Autodesk Inventor part; units mm, degrees
(part 2 of 2)
sketch "Sketch14" plane through (0, 0, 0) normal (-1, 0, 0) x (0, 0, 1)
  line L0 (-10.4499, -187.9273) -> (8.7669, -187.9273) construction
  line L1 (8.7669, -187.9273) -> (8.7669, -196.7101) construction
  line L2 (8.7669, -196.7101) -> (-10.4499, -196.7101) construction
  line L3 (-10.4499, -196.7101) -> (-10.4499, -187.9273) construction
  line L4 (-23.4175, -195.887) -> (-20.8486, -188.267)
  line L5 (-20.8486, -188.267) -> (-19.6013, -188.267)
  line L6 (-19.6013, -188.267) -> (-17.0325, -195.887)
  line L7 (-17.0325, -195.887) -> (-18.1008, -195.887)
  line L8 (-18.1008, -195.887) -> (-18.7924, -193.7566)
  line L9 (-18.7924, -193.7566) -> (-21.7008, -193.7566)
  line L10 (-21.7008, -193.7566) -> (-22.3924, -195.887)
  line L11 (-22.3924, -195.887) -> (-23.4175, -195.887)
  line L12 (-19.0702, -192.8921) -> (-20.2497, -189.3044)
  line L13 (-20.2497, -189.3044) -> (-21.4229, -192.8921)
  line L14 (-21.4229, -192.8921) -> (-19.0702, -192.8921)
  line L15 (-10.4128, -195.887) -> (-11.7281, -195.887)
  line L16 (-11.7281, -195.887) -> (-14.1364, -192.855)
  line L17 (-14.1364, -192.855) -> (-15.2973, -192.855)
  line L18 (-15.2973, -192.855) -> (-15.2973, -195.887)
  line L19 (-15.2973, -195.887) -> (-16.31, -195.887)
  line L20 (-16.31, -195.887) -> (-16.31, -188.267)
  line L21 (-16.31, -188.267) -> (-14.3463, -188.267)
  spline S0 degree 2 poles (-14.3463, -188.267) (-13.6918, -188.267) (-12.8087, -188.409) (-12.4074, -188.6683) knots 0 0 0 1 2 2 2
  spline S1 degree 2 poles (-12.4074, -188.6683) (-12.006, -188.9277) (-11.5429, -189.7366) (-11.5429, -190.3356) knots 0 0 0 1 2 2 2
  spline S2 degree 2 poles (-11.5429, -190.3356) (-11.5429, -191.1692) (-12.395, -192.2993) (-13.1237, -192.571) knots 0 0 0 1 2 2 2
  line L22 (-13.1237, -192.571) -> (-10.4128, -195.887)
  spline S3 degree 2 poles (-12.5988, -190.4159) (-12.5988, -190.0824) (-12.8334, -189.5699) (-13.0804, -189.4032) knots 0 0 0 1 2 2 2
  spline S4 degree 2 poles (-13.0804, -189.4032) (-13.2966, -189.2612) (-13.8708, -189.1438) (-14.2907, -189.1438) knots 0 0 0 1 2 2 2
  line L23 (-14.2907, -189.1438) -> (-15.2973, -189.1438)
  line L24 (-15.2973, -189.1438) -> (-15.2973, -192.009)
  line L25 (-15.2973, -192.009) -> (-14.4081, -192.009)
  spline S5 degree 2 poles (-14.4081, -192.009) (-13.9696, -192.009) (-13.2719, -191.8547) (-13.031, -191.6138) knots 0 0 0 1 2 2 2
  spline S6 degree 2 poles (-13.031, -191.6138) (-12.8087, -191.4039) (-12.5988, -190.8111) (-12.5988, -190.4159) knots 0 0 0 1 2 2 2
  line L26 (-8.0293, -195.887) -> (-8.0293, -189.1685)
  line L27 (-8.0293, -189.1685) -> (-10.5857, -189.1685)
  line L28 (-10.5857, -189.1685) -> (-10.5857, -188.267)
  line L29 (-10.5857, -188.267) -> (-4.4601, -188.267)
  line L30 (-4.4601, -188.267) -> (-4.4601, -189.1685)
  line L31 (-4.4601, -189.1685) -> (-7.0166, -189.1685)
  line L32 (-7.0166, -189.1685) -> (-7.0166, -195.887)
  line L33 (-7.0166, -195.887) -> (-8.0293, -195.887)
  spline S7 degree 2 poles (-1.564, -196.0228) (-2.3914, -196.0228) (-3.5524, -195.677) (-4.0649, -195.43) knots 0 0 0 1 2 2 2
  line L34 (-4.0649, -195.43) -> (-4.0649, -194.158)
  line L35 (-4.0649, -194.158) -> (-3.9908, -194.158)
  spline S8 degree 2 poles (-3.9908, -194.158) (-3.4906, -194.6273) (-2.2247, -195.146) (-1.6381, -195.146) knots 0 0 0 1 2 2 2
  spline S9 degree 2 poles (-1.6381, -195.146) (-0.7983, -195.146) (0.06, -194.4482) (0.06, -193.8739) knots 0 0 0 1 2 2 2
  spline S10 degree 2 poles (0.06, -193.8739) (0.06, -193.417) (-0.3907, -192.8489) (-0.8786, -192.7068) knots 0 0 0 1 2 2 2
  spline S11 degree 2 poles (-0.8786, -192.7068) (-1.2305, -192.608) (-1.8172, -192.4722) (-2.2556, -192.361) knots 0 0 0 1 2 2 2
  spline S12 degree 2 poles (-2.2556, -192.361) (-2.6508, -192.256) (-3.2745, -191.9411) (-3.5153, -191.6879) knots 0 0 0 1 2 2 2
  spline S13 degree 2 poles (-3.5153, -191.6879) (-3.75, -191.4348) (-4.0093, -190.7555) (-4.0093, -190.3109) knots 0 0 0 1 2 2 2
  spline S14 degree 2 poles (-4.0093, -190.3109) (-4.0093, -189.3847) (-2.5643, -188.1311) (-1.4467, -188.1311) knots 0 0 0 1 2 2 2
  spline S15 degree 2 poles (-1.4467, -188.1311) (-0.8045, -188.1311) (0.3317, -188.3843) (0.8196, -188.6251) knots 0 0 0 1 2 2 2
  line L36 (0.8196, -188.6251) -> (0.8196, -189.8354)
  line L37 (0.8196, -189.8354) -> (0.7455, -189.8354)
  spline S16 degree 2 poles (0.7455, -189.8354) (0.3811, -189.502) (-0.7551, -189.008) (-1.3787, -189.008) knots 0 0 0 1 2 2 2
  spline S17 degree 2 poles (-1.3787, -189.008) (-2.0827, -189.008) (-2.9534, -189.6687) (-2.9534, -190.2059) knots 0 0 0 1 2 2 2
  spline S18 degree 2 poles (-2.9534, -190.2059) (-2.9534, -190.6876) (-2.4408, -191.2619) (-1.9592, -191.3915) knots 0 0 0 1 2 2 2
  spline S19 degree 2 poles (-1.9592, -191.3915) (-1.6381, -191.478) (-0.7057, -191.7003) (-0.3969, -191.7929) knots 0 0 0 1 2 2 2
  spline S20 degree 2 poles (-0.3969, -191.7929) (0.3873, -192.0337) (1.116, -193.0032) (1.116, -193.7134) knots 0 0 0 1 2 2 2
  spline S21 degree 2 poles (1.116, -193.7134) (1.116, -194.1641) (0.7516, -195.0286) (0.4244, -195.3312) knots 0 0 0 1 2 2 2
  spline S22 degree 2 poles (0.4244, -195.3312) (0.06, -195.6647) (-0.8662, -196.0228) (-1.564, -196.0228) knots 0 0 0 1 2 2 2
  line L38 (4.7222, -193.0156) -> (1.8385, -193.0156)
  line L39 (1.8385, -193.0156) -> (1.8385, -192.0893)
  line L40 (1.8385, -192.0893) -> (4.7222, -192.0893)
  line L41 (4.7222, -192.0893) -> (4.7222, -193.0156)
  line L42 (10.3662, -195.887) -> (5.951, -195.887)
  line L43 (5.951, -195.887) -> (5.951, -188.267)
  line L44 (5.951, -188.267) -> (6.9637, -188.267)
  line L45 (6.9637, -188.267) -> (6.9637, -194.9854)
  line L46 (6.9637, -194.9854) -> (10.3662, -194.9854)
  line L47 (10.3662, -194.9854) -> (10.3662, -195.887)
  spline S23 degree 2 poles (14.275, -195.2818) (14.1577, -195.3683) (13.7625, -195.677) (13.5772, -195.7696) knots 0 0 0 1 2 2 2
  spline S24 degree 2 poles (13.5772, -195.7696) (13.324, -195.9055) (12.8486, -196.0475) (12.4163, -196.0475) knots 0 0 0 1 2 2 2
  spline S25 degree 2 poles (12.4163, -196.0475) (12.0643, -196.0475) (11.4283, -195.782) (11.1875, -195.5412) knots 0 0 0 1 2 2 2
  spline S26 degree 2 poles (11.1875, -195.5412) (10.959, -195.3065) (10.6811, -194.6149) (10.6811, -194.2321) knots 0 0 0 1 2 2 2
  spline S27 degree 2 poles (10.6811, -194.2321) (10.6811, -193.6393) (11.1813, -192.7995) (11.7247, -192.5586) knots 0 0 0 1 2 2 2
  spline S28 degree 2 poles (11.7247, -192.5586) (12.2063, -192.3363) (13.5155, -192.1696) (14.275, -192.1264) knots 0 0 0 1 2 2 2
  line L48 (14.275, -192.1264) -> (14.275, -191.9411)
  spline S29 degree 2 poles (14.275, -191.9411) (14.275, -191.6077) (14.0712, -191.1939) (13.886, -191.0766) knots 0 0 0 1 2 2 2
  spline S30 degree 2 poles (13.886, -191.0766) (13.7007, -190.9593) (13.1697, -190.8852) (12.8856, -190.8852) knots 0 0 0 1 2 2 2
  spline S31 degree 2 poles (12.8856, -190.8852) (12.5522, -190.8852) (11.6506, -191.0828) (11.1998, -191.2742) knots 0 0 0 1 2 2 2
  line L49 (11.1998, -191.2742) -> (11.1442, -191.2742)
  line L50 (11.1442, -191.2742) -> (11.1442, -190.2924)
  spline S32 degree 2 poles (11.1442, -190.2924) (11.4098, -190.2183) (12.404, -190.033) (12.8918, -190.033) knots 0 0 0 1 2 2 2
  spline S33 degree 2 poles (12.8918, -190.033) (13.4846, -190.033) (14.2935, -190.2183) (14.6146, -190.4591) knots 0 0 0 1 2 2 2
  spline S34 degree 2 poles (14.6146, -190.4591) (14.9295, -190.6938) (15.2383, -191.4409) (15.2383, -191.9782) knots 0 0 0 1 2 2 2
  line L51 (15.2383, -191.9782) -> (15.2383, -195.887)
  line L52 (15.2383, -195.887) -> (14.275, -195.887)
  line L53 (14.275, -195.887) -> (14.275, -195.2818)
  line L54 (14.275, -194.4791) -> (14.275, -192.8921)
  spline S35 degree 2 poles (14.275, -192.8921) (13.9292, -192.923) (12.8856, -193.0279) (12.5583, -193.1267) knots 0 0 0 1 2 2 2
  spline S36 degree 2 poles (12.5583, -193.1267) (12.1755, -193.2441) (11.6753, -193.7319) (11.6753, -194.1641) knots 0 0 0 1 2 2 2
  spline S37 degree 2 poles (11.6753, -194.1641) (11.6753, -194.6581) (12.231, -195.1583) (12.7621, -195.1583) knots 0 0 0 1 2 2 2
  spline S38 degree 2 poles (12.7621, -195.1583) (13.2129, -195.1583) (13.9539, -194.7693) (14.275, -194.4791) knots 0 0 0 1 2 2 2
  spline S39 degree 2 poles (21.3825, -192.9353) (21.3825, -194.337) (20.024, -196.0475) (18.9989, -196.0475) knots 0 0 0 1 2 2 2
  spline S40 degree 2 poles (18.9989, -196.0475) (18.5358, -196.0475) (17.875, -195.819) (17.5539, -195.6214) knots 0 0 0 1 2 2 2
  line L55 (17.5539, -195.6214) -> (17.4922, -195.887)
  line L56 (17.4922, -195.887) -> (16.5906, -195.887)
  line L57 (16.5906, -195.887) -> (16.5906, -187.9273)
  line L58 (16.5906, -187.9273) -> (17.5539, -187.9273)
  line L59 (17.5539, -187.9273) -> (17.5539, -190.7679)
  spline S41 degree 2 poles (17.5539, -190.7679) (17.9183, -190.4406) (18.7642, -190.0083) (19.3015, -190.0083) knots 0 0 0 1 2 2 2
  spline S42 degree 2 poles (19.3015, -190.0083) (20.271, -190.0083) (21.3825, -191.5583) (21.3825, -192.9353) knots 0 0 0 1 2 2 2
  spline S43 degree 2 poles (20.3883, -193.0094) (20.3883, -191.9843) (19.7646, -190.9222) (19.073, -190.9222) knots 0 0 0 1 2 2 2
  spline S44 degree 2 poles (19.073, -190.9222) (18.684, -190.9222) (17.8812, -191.2927) (17.5539, -191.5768) knots 0 0 0 1 2 2 2
  line L60 (17.5539, -191.5768) -> (17.5539, -194.8557)
  spline S45 degree 2 poles (17.5539, -194.8557) (17.9183, -195.0348) (18.4802, -195.183) (18.8136, -195.183) knots 0 0 0 1 2 2 2
  spline S46 degree 2 poles (18.8136, -195.183) (19.5485, -195.183) (20.3883, -194.1394) (20.3883, -193.0094) knots 0 0 0 1 2 2 2
  point P0 (0, 0)
  constraints: 2 other
emboss "Emboss2" sketch "Sketch14" operation cut depth 2.54 direction (1, 0, 0)
sketch "Sketch15" plane through (0, -213.7841, 48.4212) normal (0, 0, 1) x (1, 0, 0)
  line L0 (21.59, 0) -> (21.59, 261.366) projected
  line L1 (17.272, 162.687) -> (21.59, 162.687)
  line L2 (21.59, 162.687) -> (21.59, 170.688)
  line L3 (21.59, 170.688) -> (17.272, 170.688)
  line L4 (17.272, 170.688) -> (17.272, 162.687)
  line L5 (21.59, 264.541) -> (0, 264.541) projected
  point P0 (0, 213.7841)
  point P1 (19.431, 170.688)
  dimension "d78" = 8.001
  dimension "d79" = 4.318
  dimension "d83" = 101.854
  constraints: 8 end point, 2 parallel, 1 horizontal, 1 midpoint, 1 perpendicular, 1 point on line
  measures "d78" distance of L3.end L1.start
  measures "d79" distance between parallel lines of L0 L4
  measures "d83" distance between parallel lines of L5 L1
extrude "Extrusion9" cut sketch "Sketch15" against normal blind 6.35
sketch "Sketch18" plane through (0, -216.9591, -50.0038) normal (0, -1, 0) x (1, 0, 0)
  line L0 (21.59, 43.2816) -> (21.59, 53.2892)
  line L1 (21.59, 53.2892) -> (20.3708, 53.2892)
  line L2 (20.3708, 53.2892) -> (18.6182, 51.2892)
  line L3 (18.6182, 45.2816) -> (18.6182, 51.2892)
  line L4 (21.59, 98.425) -> (0, 98.425) projected
  line L5 (21.59, 95.25) -> (21.59, 0) projected
  line L6 (21.59, 43.2816) -> (20.3708, 43.2816)
  line L7 (20.3708, 43.2816) -> (18.6182, 45.2816)
  point P0 (20.9804, 53.2892)
  dimension "d91" = 1.2192
  dimension "d92" = 2
  dimension "d94" = 6.0076
  dimension "d95" = 10.0076
  dimension "d98" = 1.7526
  dimension "d99" = 0
  dimension "d165" = 45.1358
  constraints: 12 end point, 1 horizontal, 1 midpoint
  measures "d91" distance of L0.end L1.end
  measures "d92" vertical distance of L1.end L2.end
  measures "d94" distance of L3.start L2.end
  measures "d95" distance of L0.start L0.end
  measures "d98" distance from line of L1.end L3
  measures "d99" distance between parallel lines of L5 L0
  measures "d165" distance from line of L4 point (20.98, 53.289)
extrude "Extrusion10" cut sketch "Sketch18" against normal blind 6.35
sketch "Sketch19" plane through (0, 13.9785, -4.7779) normal (-1, 0, 0) x (0, 0, 1)
  arc A0 (-41.146, 32.7145) -> (-44.2099, 29.4687) centre (-43.3209, 31.6985) ccw projected
  circle A1 centre (-43.3209, 31.6985) radius 4.5085
  arc A2 (45.9442, 32.7145) -> (49.0081, 29.4687) centre (48.1191, 31.6985) ccw projected
  circle A3 centre (48.1191, 31.6985) radius 4.5085
  circle A4 centre (-43.3209, -225.8575) radius 2.4005 projected
  circle A5 centre (-43.3209, -225.8575) radius 4.5085
  arc A6 (45.9433, -226.8716) -> (49.0081, -223.6277) centre (48.1191, -225.8575) ccw projected
  circle A7 centre (48.1191, -225.8575) radius 4.5085
  circle A8 centre (-38.2409, -77.5215) radius 4.5085
  circle A9 centre (-38.2409, -77.5215) radius 2.4005 projected
  circle A10 centre (43.0391, -77.5215) radius 4.5085
  circle A11 centre (43.0391, -77.5215) radius 2.4005 projected
  point P0 (0, 0)
  point P1 (48.9872, -224.0625)
  dimension "d110" = 9.017
  dimension "d111" = 9.017
  dimension "d112" = 9.017
  dimension "d113" = 9.017
  dimension "d120" = 9.017
  dimension "d121" = 0
  dimension "d122" = 0
  dimension "d123" = 9.017
  dimension "d124" = 0
  dimension "d125" = 0
  constraints: 6 centre point, 4 coincident
  measures "d110" diameter of A1
  measures "d111" diameter of A3
  measures "d112" diameter of A5
  measures "d113" diameter of A7
  measures "d120" diameter of A8
  measures "d121" distance of A9.centre A8.centre
  measures "d122" distance of A9.centre A8.centre
  measures "d123" diameter of A10
  measures "d124" distance of A11.centre A10.centre
  measures "d125" distance of A11.centre A10.centre
extrude "Extrusion11" cut sketch "Sketch19" against normal blind 5 contours A1 | A3 | A4 | A5 | A7 | A8 | A9 | A10 | A11
sketch "Sketch20" plane through (0, -216.9591, -50.0038) normal (0, -1, 0) x (1, 0, 0)
  circle A0 centre (19.558, 65.4174) radius 2.032
  line L0 (21.59, 98.425) -> (0, 98.425) projected
  line L1 (21.59, 95.25) -> (21.59, 53.2892) projected
  point P0 (0, 50.0038)
  dimension "d126" = 4.064
  dimension "d127" = 33.0076
  dimension "d128" = 2.032
  constraints: 1 centre point
  measures "d126" diameter of A0
  measures "d127" distance from line of L0 A0.centre
  measures "d128" distance from line of L1 A0.centre
extrude "Extrusion12" cut sketch "Sketch20" against normal blind 13.97
sketch "Sketch21" plane through (6.35, 0, 0) normal (1, 0, 0) x (0, 0, -1)
  circle A0 centre (-38.2612, -63.5431) radius 2.4005 projected
  circle A1 centre (-38.2612, -63.5431) radius 2.4005
  circle A2 centre (43.0188, -63.5431) radius 2.4005 projected
  circle A3 centre (43.0188, -63.5431) radius 1.9939
  line L0 (-35.2132, -58.3752) -> (-35.2132, -68.7109)
  line L1 (-42.0712, -70.6551) -> (-42.0712, -56.4311)
  line L2 (-36.9448, -55.5472) -> (-40.101, -53.9363)
  line L3 (-41.462, -52.597) -> (-42.0712, -51.4492)
  line L4 (-36.9448, -71.5389) -> (-40.101, -73.1498)
  line L5 (-41.462, -74.4891) -> (-42.0712, -75.6369)
  arc A4 (-41.462, -52.597) -> (-40.101, -53.9363) centre (-38.6576, -51.1084) ccw
  arc A5 (-40.101, -73.1498) -> (-41.462, -74.4891) centre (-38.6576, -75.9777) ccw
  arc A6 (-36.9448, -71.5389) -> (-35.2132, -68.7109) centre (-38.3882, -68.7109) ccw
  arc A7 (-35.2132, -58.3752) -> (-36.9448, -55.5472) centre (-38.3882, -58.3752) ccw
  line L6 (46.8288, -56.4311) -> (46.8288, -70.6551)
  line L7 (39.9708, -68.7109) -> (39.9708, -58.3752)
  line L8 (41.7024, -55.5472) -> (44.852, -53.9397)
  line L9 (46.213, -52.6004) -> (46.8288, -51.4403)
  line L10 (41.7024, -71.5389) -> (44.852, -73.1465)
  line L11 (46.213, -74.4858) -> (46.8288, -75.6459)
  arc A8 (46.213, -74.4858) -> (44.852, -73.1465) centre (43.4086, -75.9744) ccw
  arc A9 (39.9708, -68.7109) -> (41.7024, -71.5389) centre (43.1458, -68.7109) ccw
  arc A10 (44.852, -53.9397) -> (46.213, -52.6004) centre (43.4086, -51.1117) ccw
  arc A11 (41.7024, -55.5472) -> (39.9708, -58.3752) centre (43.1458, -58.3752) ccw
  line L12 (46.8288, -51.4403) -> (46.8288, -75.6459)
  line L13 (-42.0712, -51.4492) -> (-42.0712, -75.6369)
  point P0 (0, 0)
  point P1 (-37.8414, -63.5431)
  point P2 (-37.853, -70.6551)
  point P3 (-37.853, -56.4311)
  point P4 (-40.9926, -53.4812)
  point P5 (-40.9926, -73.6049)
  point P6 (43.3998, -70.6551)
  point P7 (45.7436, -53.4846)
  dimension "d135" = 14.224
  dimension "d149" = 4.801
  dimension "d168" = 145
  dimension "d169" = 145
  dimension "d170" = 117.04
  dimension "d171" = 117.04
  dimension "d172" = 2.032
  dimension "d173" = 2.032
  dimension "d175" = 3.175
  dimension "d176" = 3.1561
  dimension "d177" = 3.1561
  dimension "d179" = 7.112
  dimension "d181" = 145
  dimension "d182" = 145
  dimension "d183" = 117.04
  dimension "d184" = 117.04
  dimension "d185" = 3.175
  dimension "d187" = 3.175
  dimension "d188" = 3.1496
  dimension "d189" = 2.0443
  dimension "d190" = 3.1496
  constraints: 28 end point, 16 point on circle, 16 tangent, 10 centre point, 6 equal radius, 6 point on line, 2 coincident, 2 parallel, 2 vertical
  measures "d135" distance of point (-37.853, -70.655) point (-37.853, -56.431)
  measures "d149" diameter of A0
  measures "d168" angle of L2 L3
  measures "d169" angle of L5 L4
  measures "d170" angle of L4 L0
  measures "d171" angle of L0 L2
  measures "d172" vertical distance of point (-40.993, -53.481) L3.end
  measures "d173" vertical distance of point (-40.993, -73.605) L5.end
  measures "d175" radius of A4
  measures "d176" horizontal distance of L2.start L2.end
  measures "d177" horizontal distance of L4.start L4.end
  measures "d179" vertical distance of point (43.4, -70.655) A3.centre
  measures "d181" angle of L8 L9
  measures "d182" angle of L11 L10
  measures "d183" angle of L10 L7
  measures "d184" angle of L7 L8
  measures "d185" radius of A8
  measures "d187" radius of A10
  measures "d188" horizontal distance of L8.start L8.end
  measures "d189" vertical distance of L9.end point (45.744, -53.485)
  measures "d190" horizontal distance of L10.start L10.end
extrude "Extrusion13" add sketch "Sketch21" along normal blind 8.89 contours L0 A6 L4 A5 L5 L13 L1 L3 A4 L2 A7 | L6 L12 L11 A8 L10 A9 L7 A11 L8 A10 L9
fillet "Fillet6" radius 0.508 11 edges at (17.272, 50.7569, -22.6988) (12.954, 50.7569, -1.1088) (17.272, 50.7569, 20.4812) (19.431, -43.0961, 48.4212) (17.272, -47.0966, 48.4212) (19.431, -51.0971, 48.4212) (20.9804, -216.9591, 3.2854) (19.4945, -216.9591, 2.2854) (18.6182, -216.9591, -1.7184) (19.4945, -216.9591, -5.7222) (20.9804, -216.9591, -6.7222)
sketch "Sketch22" plane through (0, -216.9591, -50.0038) normal (0, -1, 0) x (1, 0, 0)
  line L0 (21.59, 65.4174) -> (21.59, 91.059) projected
  line L1 (13.97, 9.525) -> (21.59, 9.525)
  line L2 (21.59, 9.525) -> (21.59, 85.725)
  line L3 (21.59, 85.725) -> (13.97, 85.725)
  line L4 (13.97, 85.725) -> (13.97, 9.525)
  line L5 (21.59, 98.425) -> (0, 98.425) projected
  line L6 (0, -3.175) -> (21.59, -3.175) projected
  line L7 (10.4902, 42.7736) -> (13.97, 42.7736)
  line L8 (13.97, 42.7736) -> (13.97, 53.7972)
  line L9 (13.97, 53.7972) -> (10.4902, 53.7972)
  line L10 (10.4902, 53.7972) -> (10.4902, 42.7736)
  line L11 (21.59, 53.7972) -> (20.1405, 53.7972) projected
  line L12 (20.1405, 42.7736) -> (21.59, 42.7736) projected
  line L13 (18.1102, 51.4803) -> (18.1102, 45.0905) projected
  point P0 (0, 50.0038)
  point P1 (17.78, 85.725)
  point P2 (17.78, 9.525)
  point P3 (20.8653, 53.7972)
  point P4 (12.2301, 53.7972)
  point P5 (20.8653, 42.7736)
  point P6 (10.4902, 48.2854)
  point P7 (13.97, 42.7736)
  dimension "d191" = 12.7
  dimension "d192" = 12.7
  dimension "d193" = 0
  dimension "d194" = 0
  dimension "d195" = 7.62
  dimension "d203" = 7.62
  constraints: 16 end point, 6 midpoint, 4 parallel, 2 horizontal, 2 perpendicular, 2 point on line
  measures "d191" distance from line of L5 point (17.78, 85.725)
  measures "d192" distance from line of L6 point (17.78, 9.525)
  measures "d193" vertical distance of point (20.865, 53.797) point (12.23, 53.797)
  measures "d194" distance from line of point (20.865, 42.774) L7
  measures "d195" distance from line of L13 point (10.49, 48.285)
  measures "d203" distance between parallel lines of L2 L4
extrude "Extrusion14" cut sketch "Sketch22" against normal blind 7.62
fillet "Fillet7" radius 0.762 4 edges at (10.4902, -213.7841, 3.7934) (10.4902, -213.7841, -7.2302) (13.97, -213.7841, -7.2302) (13.97, -213.7841, 3.7934)
fillet "Fillet8" radius 0.762 11 edges at (13.7468, -216.9591, 4.0166) (12.2301, -216.9591, 3.7934) (10.7134, -216.9591, 3.5702) (10.4902, -216.9591, -1.7184) (10.7134, -216.9591, -7.007) (12.2301, -216.9591, -7.2302) (13.7468, -216.9591, -7.4534) (13.97, -216.9591, -24.2355) (13.97, -216.9591, 20.1383) (17.78, -216.9591, -40.4788) (17.78, -216.9591, 35.7212)
body "Solid1"
